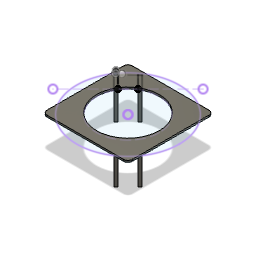
Gutter-Outlet-SensorHolder (Autodesk Fusion 360 design; units mm, degrees)
Autodesk Fusion 360 part; units mm, degrees
sketch "MainRest" plane through (0, 0, 0) normal (0, 1, 0) x (1, 0, 0)
  circle A0 centre (0, 0) radius 36 construction
  line L0 (27, 30) -> (-27, 30)
  line L1 (-30, 27) -> (-30, -27)
  line L2 (-27, -30) -> (27, -30)
  line L3 (30, -27) -> (30, 27)
  line L4 (30, 30) -> (-30, -30) construction
  line L5 (-30, 30) -> (30, -30) construction
  circle A1 centre (0, 0) radius 22
  arc A2 (-27, 30) -> (-30, 27) centre (-27, 27) ccw
  arc A3 (27, -30) -> (30, -27) centre (27, -27) ccw
  arc A4 (-30, -27) -> (-27, -30) centre (-27, -27) ccw
  arc A5 (30, 27) -> (27, 30) centre (27, 27) ccw
  dimension "d3" = 72
  dimension "d4" = 60
  dimension "d5" = 60
  dimension "d8" = 44
  dimension "d9" = 3
  constraint coincident A0.centre A1.centre
  constraint horizontal L0
  constraint perpendicular L0 L1
  constraint parallel L0 L2
  constraint parallel L1 L3
  constraint coincident L4 A0.centre
  constraint coincident L5 A0.centre
  constraint concentric A0 A1
  constraint coincident L5.start L0
  constraint coincident L5.start L1
  constraint tangent L0 A2
  constraint tangent L1 A2
  constraint coincident L5.end L2
  constraint coincident L5.end L3
  constraint tangent L2 A3
  constraint tangent L3 A3
  constraint equal A2 A3
  constraint coincident L4.end L2
  constraint coincident L4.end L1
  constraint tangent L2 A4
  constraint tangent L1 A4
  constraint equal A2 A4
  constraint coincident L4.start L3
  constraint coincident L4.start L0
  constraint tangent L3 A5
  constraint tangent L0 A5
  constraint equal A2 A5
  measures "d3" diameter of A0
  measures "d4" distance of L4.end L5.end
  measures "d5" distance of L5.start L4.end
  measures "d8" diameter of A1
  measures "d9" radius of A2
extrude "Extrude1" add sketch "MainRest" along normal blind 1.2
ref_plane "WorkPlane1" through (-15.5563, 1.9245, -15.5563) normal (0.707107, 0, 0.707107) x (-0.707107, 0, 0.707107)
ref_plane "WorkPlane2" through (15.5563, 0.9394, 15.5563) normal (-0.707107, 0, -0.707107) x (0.707107, 0, -0.707107)
sketch "SensorHolder" plane through (0, 0, 0) normal (0, -1, 0) x (1, 0, 0)
  circle A0 centre (0, 0) radius 22
  arc A1 (27, -30) -> (30, -27) centre (27, -27) ccw
  line L0 (30, -27) -> (30, 27)
  arc A2 (30, 27) -> (27, 30) centre (27, 27) ccw
  line L1 (27, 30) -> (-27, 30)
  arc A3 (-27, 30) -> (-30, 27) centre (-27, 27) ccw
  line L2 (-30, 27) -> (-30, -27)
  arc A4 (-30, -27) -> (-27, -30) centre (-27, -27) ccw
  line L3 (-27, -30) -> (27, -30)
  line L4 (10.8437, -41.9563) -> (-41.9563, 10.8437) construction
  circle A5 centre (0, 0) radius 22 construction
  arc A6 (-29.1233, -20.3743) -> (-29.4263, -20.7386) centre (-26.9042, -22.5282) ccw
  circle A7 centre (0, 0) radius 36
  line L5 (-19.0919, -12.0208) -> (-12.0208, -19.0919) construction
  line L6 (-12.0208, -19.0919) -> (-20.5061, -27.5772) construction
  line L7 (-20.5061, -27.5772) -> (-27.5772, -20.5061) construction
  line L8 (-27.5772, -20.5061) -> (-19.0919, -12.0208) construction
  line L9 (-20.5061, -27.5772) -> (-12.0208, -19.0919) construction
  line L10 (-27.5772, -20.5061) -> (-19.0919, -12.0208)
  line L11 (-19.0919, -12.0208) -> (-20.5061, -10.6066)
  line L12 (-20.5061, -10.6066) -> (-28.9914, -19.0919)
  line L13 (-28.9914, -19.0919) -> (-27.5772, -20.5061)
  line L14 (-20.5061, -27.5772) -> (-12.0208, -19.0919)
  line L15 (-12.0208, -19.0919) -> (-10.6066, -20.5061)
  line L16 (-10.6066, -20.5061) -> (-19.0919, -28.9914)
  line L17 (-19.0919, -28.9914) -> (-20.5061, -27.5772)
  point P0 (-31.1127, -22.6274)
  dimension "d62" = 10
  dimension "d63" = 12
  dimension "d65" = 2
  dimension "d66" = 2
  constraint coincident A7 A6.end
  constraint perpendicular L5 L6
  constraint parallel L5 L7
  constraint parallel L6 L8
  constraint coincident L4 L5.end
  constraint coincident L4 L5.start
  constraint midpoint L4 L5
  constraint perpendicular L10 L11
  constraint parallel L10 L12
  constraint parallel L11 L13
  constraint perpendicular L14 L15
  constraint parallel L14 L16
  constraint parallel L15 L17
  measures "d62" distance of L6 L8
  measures "d63" distance of L5 L7
  measures "d65" distance of L7.end L12.end
  measures "d66" distance of L6.end L16.end
extrude "Extrude5" add sketch "SensorHolder" along normal blind 20 contours L10 L11 L12 L13 | L14 L15 L16 L17
ref_plane "WorkPlane3" through (0, 1.9245, 0) normal (0.707107, 0, 0.707107) x (-0.707107, 0, 0.707107)
mirror "Mirror1" about plane through (0, 1.9245, 0) normal (0.707107, 0, 0.707107) of "Extrude5"
equation "GutterSquareHoleWidth = 60 mm"
equation "GutterHoleDiameter = 72 mm"
equation "d3 = GutterHoleDiameter"
equation "d4 = GutterSquareHoleWidth"
equation "d5 = GutterSquareHoleWidth"
equation "GolfBallDiameter = 43 mm"
equation "GolfHolePadding = 1 mm"
equation "d8 = GolfBallDiameter + GolfHolePadding"
equation "d9 = SquareCornerRounding"
equation "SquareCornerRounding = 3 mm"
equation "SquareBitThickness = 1.2 mm"
equation "d12 = SquareBitThickness"
equation "SensorHeight = 20 mm"
equation "SensorWidth = 10 mm"
equation "SensorDepth = 8 mm"
equation "SensorRealDepth = 12 mm" comment "Measure with the screw"
equation "SensorScrewBottomOffset = 3 mm"
equation "SensorScrewHoleDiameter = 4 mm"
equation "InsertDiameter = 4 mm"
equation "InsertHeight = 4 mm"
equation "SensorHolderThickness = 2 mm"
equation "d46 = SensorHeight"
equation "d62 = SensorWidth"
equation "d63 = SensorRealDepth"
equation "d65 = SensorHolderThickness"
equation "d66 = SensorHolderThickness"
